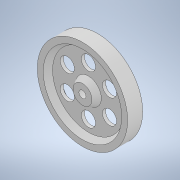
# Autodesk Inventor part: Wheel
Saved by Autodesk Inventor 2022 (Build 260153000, 153)
## iProperties
Created: 2022-08-10
Part Number: Wheel
Material: Generic
Document SubType Name: Modeling
Designer: Nick
Density: 1 g/cm^3
Appearance: Default
Mass: 115.115 g
Surface Area: 156.235 cm^2
Volume: 115.115 cm^3
Author: Nick
Autodesk Inventor part; units mm, degrees
ref_plane "YZ Plane" through (0, 0, 0) normal (1, 0, 0) x (0, 1, 0)
ref_plane "XZ Plane" through (0, 0, 0) normal (0, 1, 0) x (-1, 0, 0)
ref_plane "XY Plane" through (0, 0, 0) normal (0, 0, 1) x (1, 0, 0)
sketch "Sketch1" plane through (0, 0, 0) normal (0, 0, 1) x (1, 0, 0)
  circle A0 centre (0, 0) radius 38.1
  dimension "d0" = 76.2
  constraints: 1 centre point, 1 coincident
  measures "d0" diameter of A0
extrude "Extrusion1" add sketch "Sketch1" along normal blind 12.7
sketch "Sketch2" plane through (0, 0, 12.7) normal (0, 0, 1) x (1, 0, 0)
  circle A0 centre (0, 0) radius 3
  circle A1 centre (0, 16.2239) radius 4.4158
  circle A2 centre (10.9199, -6.1359) radius 5.0704
  circle A3 centre (-11.3359, -9.1519) radius 3.2327
  circle A4 centre (0, 0) radius 12.5 construction
  dimension "d3" = 6
  dimension "d6" = 25
  constraints: 5 centre point, 2 coincident
  measures "d3" diameter of A0
  measures "d6" diameter of A4
extrude "Extrusion2" cut sketch "Sketch2" against normal blind 25.4 contours A0
sketch "Sketch3" plane through (0, 0, 0) normal (1, 0, 0) x (0, 1, 0)
  line L0 (38.1, 12.7) -> (-38.1, 12.7) projected
  line L1 (38.1, 0) -> (-38.1, 0) projected
  line L2 (3, 12.7) -> (3, 0) projected
  line L3 (3, 0) -> (8, 0)
  line L4 (38.1, 0) -> (-38.1, 0) projected
  line L5 (8, 0) -> (10.8868, 5)
  line L6 (10.8868, 5) -> (30.2132, 5)
  line L7 (30.2132, 5) -> (33.1, 0)
  line L8 (0, -5.08) -> (0, 30.48) projected
  point P0 (0, 0)
  dimension "d8" = 120
  dimension "d9" = 5
  dimension "d10" = 5
  dimension "d11" = 5
  dimension "d13" = 120
  constraints: 8 end point, 4 point on line, 1 parallel
  measures "d8" angle of L6 L7
  measures "d9" distance of L1.start L7.end
  measures "d10" distance of L3.start L3.end
  measures "d11" distance between parallel lines of L1 L6
  measures "d13" angle of L1 L5
revolve "Revolution1" cut sketch "Sketch3" angle 360 about axis through (0, 0, -10) along (0, 0, 1) contours L1 L5 L6 L7
ref_plane "Work Plane1" through (0, 0, 6.35) normal (0, 0, -1) x (-1, 0, 0)
mirror "Mirror1" about plane through (0, 0, 6.35) normal (0, 0, -1) of "Revolution1"
sketch "Sketch4" plane through (0, 0, 5) normal (0, 0, -1) x (-1, 0, 0)
  circle A0 centre (0, 20.55) radius 6
  circle A1 centre (0, 0) radius 10.8868 projected
  circle A2 centre (0, 0) radius 30.2132 projected
  circle A3 centre (0, 0) radius 10.8868 construction
  line L0 (0, 10.8868) -> (0, 30.2132) construction
  dimension "d14" = 12
  constraints: 2 end point, 2 vertical alignment, 1 centre point, 1 coincident, 1 midpoint, 1 point on line, 1 vertical, 2 other
  measures "d14" diameter of A0
extrude "Extrusion3" cut sketch "Sketch4" against normal through all contours A0
pattern_circular "Circular Pattern1" count 6 over 360 about axis through (0, 0, 0) along (0, 0, 1) of "Extrusion3"
body "Solid1"
